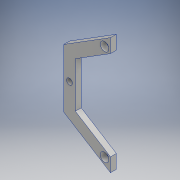
# Autodesk Inventor part: bogie
Saved by Autodesk Inventor 2018.1 (Build 221171000, 171)
## iProperties
Created: 2017-10-26
Part Number: bogie
Material: アルミニウム 6061
Document SubType Name: Modeling
Designer: Kakeru Yamashita
Density: 2.7 g/cm^3
Appearance: アルミニウム - フラット
Author: Kakeru Yamashita
Autodesk Inventor part; units mm, degrees
ref_plane "YZ Plane" through (0, 0, 0) normal (1, 0, 0) x (0, 1, 0)
ref_plane "XZ Plane" through (0, 0, 0) normal (0, 1, 0) x (-1, 0, 0)
ref_plane "XY Plane" through (0, 0, 0) normal (0, 0, 1) x (1, 0, 0)
sketch "スケッチ1" plane through (0, 0, 0) normal (0, 1, 0) x (-1, 0, 0)
  line L0 (48, 0) -> (-8, 0) projected
  line L1 (0, -70) -> (0, 70) projected
  line L2 (40, 0) -> (40, -25)
  line L3 (40, -25) -> (0, -50)
  line L4 (0, -38.2075) -> (30, -19.4575)
  line L5 (30, -19.4575) -> (30, 0)
  line L6 (40, 0) -> (40, 25)
  line L7 (40, 25) -> (0, 50)
  line L8 (0, 38.2075) -> (30, 19.4575)
  line L9 (30, 19.4575) -> (30, 0)
  line L10 (0, 50) -> (0, 38.2075)
  line L11 (0, -38.2075) -> (0, -50)
  point P0 (0, 0)
  dimension "d0" = 10
  dimension "d1" = 25
  dimension "d2" = 50
  dimension "d4" = 10
  dimension "d5" = 30
  constraints: 20 end point, 4 point on line, 4 symmetric about line, 2 collinear, 2 perpendicular, 1 parallel
  measures "d0" distance between parallel lines of L5 L2
  measures "d1" distance of L2.start L2.end
  measures "d2" vertical distance of L3.end L2.start
  measures "d4" distance between parallel lines of L3 L4
  measures "d5" distance between parallel lines of L1 L5
extrude "押し出し1" add sketch "スケッチ1" along normal blind 5 contours L2 L3 L1 L4 L5 L0 | L0 L9 L8 L1 L7 L6
sketch "スケッチ2" plane through (0, 5, 0) normal (0, 1, 0) x (1, 0, 0)
  circle A0 centre (-5, -40.9788) radius 3.75
  line L0 (0, -50) -> (0, -38.2075) projected
  line L1 (-40, -25) -> (0, -50) projected
  line L2 (-48, 0) -> (8, 0) projected
  circle A1 centre (-5, 40.9788) radius 3.75
  circle A2 centre (-35, 0) radius 2.5
  line L3 (-30, -19.4575) -> (-30, 19.4575) projected
  point P0 (0, 0)
  dimension "d8" = 7.5
  dimension "d9" = 5
  dimension "d10" = 5
  dimension "d11" = 5
  dimension "d12" = 5
  constraints: 3 centre point, 1 point on line, 1 symmetric about line, 1 other
  measures "d8" diameter of A0
  measures "d9" distance from line of L0 A0.centre
  measures "d10" distance from line of L1 A0.centre
  measures "d11" diameter of A2
  measures "d12" distance from line of L3 A2.centre
extrude "押し出し2" cut sketch "スケッチ2" against normal blind 5
